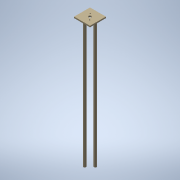
# Autodesk Inventor part: Shield_1
Saved by Autodesk Inventor 2020 (Build 240168000, 168)
## iProperties
Created: 2015-02-10
Part Number: Shield_1
Material: Generic
Document SubType Name: Modeling
Designer: Pascal
Density: 1 g/cm^3
Appearance: Beige
Author: Pascal
Autodesk Inventor part; units mm, degrees
ref_plane "YZ Plane" through (0, 0, 0) normal (1, 0, 0) x (0, 1, 0)
ref_plane "XZ Plane" through (0, 0, 0) normal (0, 1, 0) x (-1, 0, 0)
ref_plane "XY Plane" through (0, 0, 0) normal (0, 0, 1) x (1, 0, 0)
sketch "Sketch1" plane through (0, 0, 0) normal (0, 1, 0) x (-1, 0, 0)
  line L0 (19.05, 19.05) -> (-19.05, 19.05)
  line L1 (-19.05, 19.05) -> (-19.05, -19.05)
  line L2 (-19.05, -19.05) -> (19.05, -19.05)
  line L3 (19.05, -19.05) -> (19.05, 19.05)
  point P0 (0, 0)
  dimension "d0" = 38.1
  dimension "d1" = 38.1
  dimension "d77" = 19.05
  dimension "d78" = 19.05
  constraints: 8 end point, 2 parallel, 1 horizontal, 1 perpendicular
  measures "d0" distance of L1.end L2.end
  measures "d1" distance of L2.end L0.start
  measures "d77" distance from line of L3 point (0, 0)
  measures "d78" distance from line of L2 point (0, 0)
extrude "Extrusion1" add sketch "Sketch1" along normal blind 3.175
hole "Hole5" at (-6.35, 3.175, -7.1374) direction (0, -1, 0) diameter 2.54 depth 3.175
hole "Hole6" at (6.35, 3.175, 7.1437) direction (0, -1, 0) diameter 2.54 depth 3.175
sketch "Sketch2" plane through (0, 3.175, 0) normal (0, 1, 0) x (1, 0, 0)
  circle A0 centre (0, 0) radius 3.175
  dimension "d58" = 6.35
  constraints: 1 centre point, 1 coincident
  measures "d58" diameter of A0
extrude "Extrusion2" cut sketch "Sketch2" against normal blind 304.8
sketch "Sketch7" plane through (0, 3.175, 0) normal (0, 1, 0) x (1, 0, 0)
  circle A0 centre (0, 0) radius 19.05
  circle A1 centre (0, 12.7) radius 3.175
  circle A2 centre (0, 0) radius 12.7
  circle A3 centre (0, 0) radius 3.175
  circle A4 centre (-12.7, 0) radius 3.175
  circle A5 centre (0, -12.7) radius 3.175
  circle A6 centre (12.7, 0) radius 3.175
  dimension "d71" = 38.1
  dimension "d72" = 6.35
  dimension "d73" = 25.4
  dimension "d74" = 12.7
  dimension "d75" = 6.35
  dimension "d76" = 360
  constraints: 7 centre point, 3 coincident, 9 other
  measures "d71" diameter of A0
  measures "d72" diameter of A1
  measures "d73" diameter of A2
  measures "d74" distance of A1.centre point (0, 0)
  measures "d75" diameter of A3
extrude "Extrusion7" add sketch "Sketch7" against normal blind 304.8 contours A1 A2 | A2 A1 | A4 A2 | A2 A4 | A6 A2 | A2 A6 | A5 A2 | A2 A5
body "Solid1"
